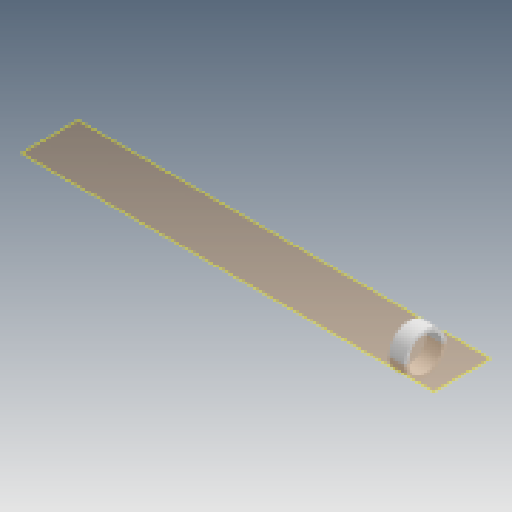
# Autodesk Inventor part: 高速轴套筒2
Saved by Autodesk Inventor 2025 (Build 290162000, 162)
## iProperties
Created: 2025-03-20
Part Number: 高速轴套筒2
Material: 常规
Document SubType Name: Modeling
Designer: liukan
Density: 1 g/cm^3
Appearance: 默认
Author: liukan
Autodesk Inventor part; units mm, degrees
ref_plane "YZ Plane" through (0, 0, 0) normal (1, 0, 0) x (0, 1, 0)
ref_plane "XZ Plane" through (0, 0, 0) normal (0, 1, 0) x (-1, 0, 0)
ref_plane "XY Plane" through (0, 0, 0) normal (0, 0, 1) x (1, 0, 0)
ref_plane "工作平面2" through (-456.5336, 175.9298, -74.6507) normal (0, 1, -0.0013) x (-1, 0, 0)
sketch "草图1" plane through (-456.5336, 175.9298, -74.6507) normal (0, 1, -0.0013) x (-1, 0, 0)
  line L0 (-309, -20.6) -> (-309, 20.6) projected
  line L1 (-294.5, 20) -> (-294.5, -20) projected
  line L2 (-295, -15) -> (-295, 15) projected
  line L3 (-295, 15) -> (-309, 15)
  line L4 (-309, 15) -> (-309, 18)
  line L5 (-309, 18) -> (-295, 18)
  line L6 (-295, 18) -> (-295, 15)
  line L7 (-294.5, 0) -> (-309, 0)
  point P0 (-456.5336, 74.4134)
  point P1 (-301.75, 0)
  point P2 (-309, 15)
  dimension "d0" = 18
  constraints: 10 end point, 3 midpoint, 2 parallel, 1 horizontal, 1 perpendicular, 1 point on line
  measures "d0" distance from line of point (-301.75, 0) L5
revolve "旋转1" add sketch "草图1" angle 360 about axis through (-162.0336, 175.9298, -74.6507) along (1, 0, 0) contours L0 L5 L6 L3
